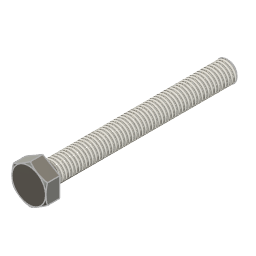
Pulley Expansion Mechanisms (Autodesk Fusion 360 archive; units mm, degrees)
design "Hexagon Head Screw ISO 4018 - M8 x 70 Steel 4.6 Plain"
description: Hexagon Head Screw ISO 4018 - M8 x 70
part number: ISO 4018 - M8 x 70 Steel 4.6 Plain
Autodesk Fusion 360 part; units mm, degrees
sketch "Sketch1" plane through (0, 0, 0) normal (0, 1, 0) x (1, 0, 0)
  line L0 (-4, 0) -> (-4, 70)
  line L1 (-4, 70) -> (0, 70)
  line L2 (0, 70) -> (0, -5.3)
  line L3 (-4, 0) -> (-7.4282, 0)
  line L4 (-7.4282, 0) -> (-7.4282, -4.689)
  line L5 (-6.37, -5.3) -> (0, -5.3)
  line L6 (-7.4282, -4.689) -> (-6.37, -5.3)
  dimension "d81" = 14.8564
  dimension "d135" = 8
  dimension "d139" = 5.3
  dimension "d140" = 70
  dimension "d156" = 12.74
  dimension "d158" = 30
  constraint perpendicular L0 L1
  constraint collinear origin L1.end L2.end
  constraint perpendicular L0 L3
  constraint coincident origin L3
  constraint vertical L2
  constraint coincident L2 L5.end
  constraint coincident L0.start L3.start
  constraint coincident L0.end L1.start
  constraint vertical L4
  measures "d139" distance of L3 L5
  measures "d140" distance of L1 L3
  measures "d158" angle of L5 L6
revolve "Revolve1" add sketch "Sketch1" angle 360 about axis through (0, 0, -70) along (0, 0, 1)
sketch "Sketch8" plane through (0, 0, 5.3) normal (0, 0, 1) x (1, 0, 0)
  circle A0 centre (0, 0) radius 7.4282
  line L0 (-6.433, -3.7141) -> (0, -7.4282)
  line L1 (0, -7.4282) -> (6.433, -3.7141)
  line L2 (6.433, -3.7141) -> (6.433, 3.7141)
  line L3 (6.433, 3.7141) -> (0, 7.4282)
  line L4 (0, 7.4282) -> (-6.433, 3.7141)
  line L5 (-6.433, 3.7141) -> (-6.433, -3.7141)
  constraint coincident A0 L0.start
  constraint coincident A0.centre origin
  constraint vertical L5
extrude "Extrude5" cut sketch "Sketch8" against normal blind 5.3 contours A0 L2 | A0 L3 | A0 L1 | A0 L4 | A0 L0 | A0 L5
fillet "Fillet7" radius 0.4 1 edges at (-3.7293, 1.4465, 0)
thread "Thread4" "ISO Metric profile 8.0 M8x1.25 M8x1.25 6g" major diameter 7.866 minor diameter 6.4455 pitch 1.25 angle 60 resizes the face on face at (-3.995, 0.1994, -46.8) from (0, 0, -2.5) to (0, 0, -70)
sketch "Sketch13" plane through (0, 0, 0) normal (0, 1, 0) x (1, 0, 0)
  line L0 (0, 70) -> (0, -5.3) construction
  line L1 (0, 70) -> (-4.08, 70)
  line L2 (-4.08, 70) -> (-4.08, 69.2)
  line L3 (-4.08, 69.2) -> (-3.2, 70)
  dimension "d160" = 0.8
  dimension "d161" = 3.2
  dimension "d162" = 4.08
  constraint coincident L0.start L1.start
  constraint perpendicular L0 L1
  constraint perpendicular L1 L2
  constraint coincident L1 L3.end
  measures "d160" distance of L1 L2.end
  measures "d161" distance of L0 L3.end
  measures "d162" distance of L0.start L2
revolve "Revolve4" cut sketch "Sketch13" angle 360 about axis through (0, 0, 1.75) along (0, 0, 1)
equation "adsk_nomlen = 70.00 mm"
equation "adsk_headh = 5.30 mm"
equation "adsk_headdia = 14.8564 mm"
equation "adsk_nomdia = 8.00 mm"
equation "d81 = adsk_headdia"
equation "d89 = -adsk_headh"
equation "adsk_waflat = 13.00 mm"
equation "adsk_thrlen = 67.50 mm"
equation "adsk_midfillet = 0.40 mm"
equation "d135 = adsk_nomdia"
equation "d139 = adsk_headh"
equation "d140 = adsk_nomlen"
equation "d142 = adsk_midfillet"
equation "adsk_endpointdia = adsk_nomdia - adsk_startlen * 2"
equation "adsk_startlen = 0.1 * adsk_nomdia"
equation "d156 = adsk_waflat * 0.98"
equation "d158 = adsk_chamang2"
equation "adsk_chamang2 = 30.00 deg"
equation "d160 = adsk_startlen"
equation "d161 = adsk_endpointdia / 2"
equation "d162 = adsk_nomdia * 0.51"
equation "d166 = min(adsk_thrlen; adsk_nomlen - adsk_midfillet - 0.001 mm)"

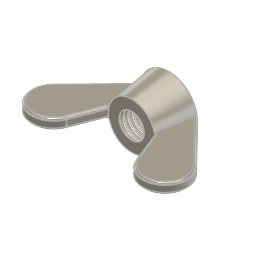
design "Wing Nut NF E27-454 - M8 Steel 6 Plain"
description: Wing Nut NF E27-454 - M8
part number: NF E27-454 - M8 Steel 6 Plain
Autodesk Fusion 360 part; units mm, degrees
sketch "Sketch1" plane through (0, 0, 0) normal (0, 1, 0) x (1, 0, 0)
  line L0 (0, 0) -> (0, -22)
  line L1 (0, -22) -> (21, -22) construction
  line L2 (21, -22) -> (21, 0) construction
  line L3 (0, 0) -> (7.75, 0)
  line L4 (0, -10) -> (6.25, -10)
  line L5 (6.25, -10) -> (7.75, 0)
  line L6 (4, 0) -> (4, -10)
  line L7 (15, -22) -> (15, -16) construction
  line L8 (21, -16) -> (15, -16) construction
  circle A0 centre (15, -16) radius 6
  line L9 (7.75, 0) -> (21, -13.554558)
  line L10 (6.25, -10) -> (10.885714, -22)
  point P0 (15, -22)
  point P1 (21, -16)
  dimension "d12" = 15.5
  dimension "d13" = 12.5
  dimension "d34" = 12
  dimension "d43" = 10
  dimension "d44" = 42
  dimension "d45" = 6
  dimension "d46" = 6
  dimension "d47" = 8
  dimension "d48" = 22
  constraint coincident L0.start L3.start
  constraint vertical L0
  constraint perpendicular L0 L3
  constraint coincident L0 L4.start
  constraint coincident L2.end L3
  constraint coincident L3 L6.start
  constraint coincident L4 L6.end
  constraint coincident L1 P0
  constraint coincident L2 P1
  constraint coincident P0 L7.start
  constraint coincident P1 L8.start
  constraint coincident L7.end L8.end
  constraint tangent A0 L10
  constraint tangent A0 L9
  measures "d34" diameter of A0
  measures "d43" distance of L3 L4
  measures "d45" distance of L2 L7
  measures "d46" distance of L1 L8
  measures "d48" distance of L1 L3
extrude "Extrude1" add sketch "Sketch1" along normal mid plane 2.8 contours L0 L3 L4 L6 | L3 L4 L5 L6 | L5 A0 L9 L10 | A0 picked at (1.333333, -3.333333) picked at (6, -3.333333) picked at (8.708979, -6.910866) picked at (15.195543, -14.265264)
mirror "Mirror1" about plane through (0, 0, 0) normal (1, 0, 0) of bodies 1 merged
revolve "Revolve1" add sketch "Sketch1" angle 360 about axis through (0, 0, 0) along (0, 0, 1) contours L0 L3 L4 L6 | L3 L4 L5 L6 picked at (1.333333, -3.333333) picked at (6, -3.333333)
revolve "Revolve2" cut sketch "Sketch1" angle 360 about axis through (0, 0, 0) along (0, 0, 1) contours L0 L3 L4 L6 picked at (1.333333, -3.333333)
thread "Thread1" "ISO Metric profile 8.0 M8x1.25 M8x1.25 6H" major diameter 8.17 minor diameter 6.7795 pitch 1.25 angle 60 resizes the face on face at (3.995028, -0.199384, 3.333333)
chamfer "Chamfer1" distance 0.8 angle 30 1 edges at (-3.160357, -1.225786, 0) measured on face at (6.211583, 0, 0)
fillet "Fillet2" radius 0.56 12 edges at (7.826564, 1.4, 14.08109) (18.244593, 1.4, 21.04704) (13.520285, 1.4, 5.902918) (-7.826564, 1.4, 14.08109) (-18.244593, 1.4, 21.04704) (-13.520285, 1.4, 5.902918) (-13.520285, -1.4, 5.902918) (-18.244593, -1.4, 21.04704) (-7.826564, -1.4, 14.08109) (13.520285, -1.4, 5.902918) (18.244593, -1.4, 21.04704) (7.826564, -1.4, 14.08109)
equation "adsk_nomdia = 8.00 mm"
equation "adsk_beardia = 15.50 mm"
equation "adsk_topdia = 12.50 mm"
equation "adsk_baseh = 10.00 mm"
equation "adsk_nheig = 22.00 mm"
equation "adsk_maxdia = 42.00 mm"
equation "adsk_wradtop = 6.00 mm"
equation "adsk_wingwidth = 2.80 mm"
equation "d12 = adsk_beardia"
equation "d13 = adsk_topdia"
equation "d16 = adsk_wingwidth"
equation "d24 = 0.1 * adsk_nomdia"
equation "d34 = adsk_wradtop * 2"
equation "d36 = 0.2 * adsk_wingwidth"
equation "d43 = adsk_baseh"
equation "d44 = adsk_maxdia"
equation "d45 = adsk_wradtop"
equation "d46 = adsk_wradtop"
equation "d47 = adsk_nomdia"
equation "d48 = adsk_nheig"
